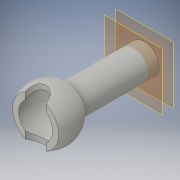
# Autodesk Inventor part: Aidan Sherry Caster
Saved by Autodesk Inventor 2016 (Build 200138000, 138)
## iProperties
Created: 2016-10-18
Part Number: Aidan Sherry Caster
Material: Generic
Document SubType Name: Modeling
Designer: sherra
Density: 1 g/cm^3
Appearance: Default
Author: sherra
Autodesk Inventor part; units mm, degrees
ref_plane "YZ Plane" through (0, 0, 0) normal (1, 0, 0) x (0, 1, 0)
ref_plane "XZ Plane" through (0, 0, 0) normal (0, 1, 0) x (-1, 0, 0)
sketch "Sketch1" plane through (0, 0, 0) normal (0, 0, 1) x (1, 0, 0)
  circle A0 centre (0, 0) radius 6.2357
  dimension "d0" = 12.4714
  constraints: 1 centre point, 1 coincident
  measures "d0" diameter of A0
extrude "Extrusion1" add sketch "Sketch1" along normal blind 40.7416
sketch "Sketch2" plane through (0, 0, 40.7416) normal (0, 0, 1) x (1, 0, 0)
  circle A0 centre (0, 0) radius 6.2357 projected
  arc A1 (-11.0871, 0) -> (11.0871, 0) centre (0, 0) ccw
  line L0 (-11.0871, 0) -> (11.0871, 0)
  dimension "d3" = 22.1742
  constraints: 2 end point, 2 point on circle, 1 centre point, 1 coincident, 1 horizontal
  measures "d3" diameter of A1
revolve "Revolution1" add sketch "Sketch2" angle 360 about axis through (-11.0871, 0, 40.7416) along (1, 0, 0) picked at (-0.499, -2.9095) contours L0 A1 A0 | A0 L0
sketch "Sketch3" plane through (0, 0, 0) normal (0, 0, -1) x (-1, 0, 0)
  point P0 (0, 0)
sketch "Sketch4" plane through (0, 0, 0) normal (0, 1, 0) x (-1, 0, 0)
  line L0 (-11.0871, 40.7416) -> (11.0871, 40.7416)
  arc A0 (0, 49.6729) -> (0, 31.8103) centre (0, 40.7416) ccw
  line L1 (0, 49.6729) -> (0, 31.8103)
  line L2 (-6.2357, 31.5743) -> (6.2357, 31.5743) projected
  point P0 (0, 0)
  constraints: 2 end point, 2 horizontal, 2 point on circle, 1 centre point, 1 midpoint, 1 vertical alignment, 2 other
revolve "Revolution2" cut sketch "Sketch4" angle 360 about axis through (0, 0, 49.6729) along (0, 0, -1)
ref_plane "Work Plane2" through (0, 0, 46.0375) normal (0, 0, 1) x (1, 0, 0)
sketch "Sketch6" plane through (0, 0, 0) normal (0, 0, 1) x (1, 0, 0)
  point P0 (0, 0)
sketch "Sketch7" plane through (0, 0, 46.0375) normal (0, 0, 1) x (1, 0, 0)
  circle A0 centre (0, 0) radius 172.7219
  line L0 (0, 172.7219) -> (0, -172.7219)
  constraints: 2 end point, 2 point on circle, 1 centre point, 1 coincident, 1 vertical
revolve "Revolution3" cut sketch "Sketch7" angle 180 about axis through (0, 172.7219, 46.0375) along (0, 1, 0) picked at (-83.5431, 10.0779) contours L0 A0
sketch "Sketch8" plane through (0, 0, 0) normal (0, 1, 0) x (-1, 0, 0)
  line L0 (7.1918, 46.0375) -> (-7.1918, 46.0375) projected
  circle A0 centre (0, 46.0375) radius 4.4094
  point P0 (0, 0)
  constraints: 1 centre point, 1 midpoint
extrude "Extrusion2" cut sketch "Sketch8" along normal mid plane 64970.025
sketch "Sketch9" plane through (0, 0, 0) normal (0, 0, -1) x (-1, 0, 0)
  circle A0 centre (0, 0) radius 3.175
  dimension "d10" = 6.35
  constraints: 1 centre point, 1 coincident
  measures "d10" diameter of A0
ref_plane "Work Plane3" through (0, 0, 4.699) normal (0, 0, 1) x (1, 0, 0)
sketch "Sketch10" plane through (0, 0, 4.699) normal (0, 0, 1) x (1, 0, 0)
  circle A0 centre (0, 0) radius 2.921
  dimension "d12" = 5.842
  constraints: 1 centre point, 1 coincident
  measures "d12" diameter of A0
loft "Loft1" cut profiles "Sketch9", "Sketch10"
body "Solid1"
